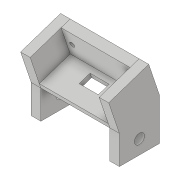
# Autodesk Inventor part: Lidar Sensor Case v3
Saved by Autodesk Inventor 2018.3 (Build 223284000, 284)
## iProperties
Created: 2019-02-04
Part Number: Lidar Sensor Case v3
Material: Generic
Document SubType Name: Modeling
Designer: aye06091
Mass: 24.5359 g
Surface Area: 111.529 cm^2
Volume: 24.5359 cm^3
Density: 1 g/cm^3
Appearance: Default
Author: aye06091
Autodesk Inventor part; units mm, degrees
ref_plane "YZ Plane" through (0, 0, 0) normal (1, 0, 0) x (0, 1, 0)
ref_plane "XZ Plane" through (0, 0, 0) normal (0, 1, 0) x (-1, 0, 0)
sketch "Sketch8" plane through (0, 0, 0) normal (1, 0, 0) x (0, 1, 0)
  line L0 (-3.8078, 7.851) -> (3.0591, -12.6251)
  line L1 (-0.2897, -12.6251) -> (-4.6863, 0.485)
  line L2 (3.0591, -12.6251) -> (-0.2897, -12.6251)
  line L3 (-4.6863, 0.485) -> (-6.818, 6.8414)
  line L4 (-3.8078, 7.851) -> (-6.818, 6.8414)
  point P0 (0, 0)
  dimension "d149" = 21.5968
  dimension "d150" = 3.175
  dimension "d151" = 3.3488
  constraints: 10 end point, 1 horizontal, 1 perpendicular
  measures "d149" distance of L0.start L0.end
  measures "d150" distance of L0.start L3.end
  measures "d151" distance of L0.end L1.start
extrude "Extrusion6" add sketch "Sketch8" along normal blind 45.72
sketch "Sketch11" plane through (0, 0, 0) normal (-1, 0, 0) x (0, 0, 1)
  line L0 (0.485, -4.6863) -> (-12.6251, -0.2897) projected
  line L1 (6.8422, -6.8159) -> (6.835, -6.8159)
  line L2 (-12.6251, -0.2897) -> (0.485, -4.6863)
  line L3 (7.851, -3.8078) -> (-12.6251, 3.0591) projected
  line L4 (13.9082, 14.2533) -> (7.851, -3.808)
  line L5 (7.851, -3.808) -> (-18.639, 5.076)
  line L6 (-18.639, 5.076) -> (-12.5817, 23.1373)
  line L7 (-12.5817, 23.1373) -> (13.9082, 14.2533)
  line L8 (-12.6251, -0.2897) -> (6.8414, -6.818) projected
  line L9 (6.8414, -6.818) -> (7.851, -3.8078) projected
  point P0 (0, 0)
  dimension "d73" = 27.94
  dimension "d76" = 0
  dimension "d88" = 19.05
  constraints: 12 end point, 2 parallel, 2 point on line, 1 perpendicular
  measures "d73" distance of L6.end L4.start
  measures "d76" distance from line of L3 L5.end
  measures "d88" distance of L5.end L6.end
extrude "Extrusion8" add sketch "Sketch11" along normal blind 6.35 contours L3 L5 L6 L7 L4
sketch "Sketch13" plane through (0, -3.8078, 7.851) normal (0, 0.9481042, 0.3179598) x (1, 0, 0)
  line L0 (0, 0) -> (0, 21.5968) projected
  line L1 (16.51, 18.0408) -> (29.21, 18.0408)
  line L2 (29.21, 18.0408) -> (29.21, 10.4208)
  line L3 (29.21, 10.4208) -> (16.51, 10.4208)
  line L4 (16.51, 10.4208) -> (16.51, 18.0408)
  point P0 (0, 8.6543)
  dimension "d55" = 7.62
  dimension "d56" = 12.7
  dimension "d57" = 16.51
  constraints: 8 end point, 2 parallel, 1 horizontal, 1 perpendicular
  measures "d55" distance of L3.end L1.start
  measures "d56" distance of L2.end L3.end
  measures "d57" distance between parallel lines of L0 L4
extrude "Extrusion10" cut sketch "Sketch13" against normal blind 25.4
sketch "Sketch15" plane through (0, 0, 0) normal (1, 0, 0) x (0, 0, -1)
  line L0 (6.5678, 21.1205) -> (12.5883, 23.1395)
  line L1 (12.5883, 23.1395) -> (18.6455, 5.0782)
  line L2 (18.6455, 5.0782) -> (12.6251, 3.0591)
  line L3 (12.6251, 3.0591) -> (6.5678, 21.1205)
  dimension "d67" = 6.35
  dimension "d69" = 0
  dimension "d70" = 0
  dimension "d87" = 19.05
  constraints: 8 end point, 2 parallel, 1 perpendicular
  measures "d67" distance of L0.start L0.end
  measures "d69" distance of point (12.625, 3.059) L2.end
  measures "d70" distance of point (12.625, 3.059) L2.end
  measures "d87" distance of L2.end L0.start
extrude "Extrusion11" add sketch "Sketch15" along normal blind 45.72
sketch "Sketch17" plane through (45.72, 0, 0) normal (1, 0, 0) x (0, 0, -1)
  line L0 (-7.851, -3.808) -> (-13.9082, 14.2533) projected
  line L1 (-7.851, -3.808) -> (-13.9082, 14.2533)
  line L2 (-13.9082, 14.2533) -> (12.5883, 23.1395)
  line L3 (12.5883, 23.1395) -> (18.6456, 5.0782)
  line L4 (18.6456, 5.0782) -> (-7.851, -3.808)
  point P0 (0, 0)
  constraints: 8 end point, 2 parallel, 1 perpendicular
extrude "Extrusion12" add sketch "Sketch17" along normal blind 6.35
sketch "Sketch19" plane through (45.72, 5.0782, -18.6456) normal (0, -0.9481019, -0.3179666) x (1, 0, 0)
  line L0 (0, 6.3501) -> (0, 0.0001) projected
  line L1 (6.35, 27.947) -> (0, 27.947)
  line L2 (0, 27.947) -> (0, 0.0001)
  line L3 (0, 0.0001) -> (6.35, 0.0001)
  line L4 (6.35, 0.0001) -> (6.35, 27.947)
  line L5 (-45.72, 6.3501) -> (0, 6.3501) projected
  line L6 (0, 0.0001) -> (0, 0.0001)
  line L7 (0, 0.0001) -> (0, 6.3501)
  line L8 (0, 6.3501) -> (0, 6.3501)
  line L9 (0, 6.3501) -> (0, 0.0001)
  line L10 (-45.72, 0.007) -> (-52.07, 0.007) projected
  line L11 (-52.07, 0.007) -> (-45.72, 0.007)
  line L12 (-45.72, 0.007) -> (-45.72, 27.947)
  line L13 (-45.72, 27.947) -> (-52.07, 27.947)
  line L14 (-52.07, 27.947) -> (-52.07, 0.007)
  point P0 (-45.72, 19.2926)
  constraints: 24 end point, 6 equal length, 3 horizontal, 3 perpendicular, 1 point on line
extrude "Extrusion13" add sketch "Sketch19" along normal blind 3.175
sketch "Sketch20" plane through (0, 5.0782, -18.6455) normal (0, -0.9481019, -0.3179666) x (1, 0, 0)
  line L0 (45.72, 0) -> (0, 0)
  line L1 (0, 0) -> (0, 6.35)
  line L2 (0, 6.35) -> (45.72, 6.35)
  line L3 (45.72, 6.35) -> (45.72, 0)
  point P0 (0, 19.2926)
  constraints: 8 end point, 2 parallel, 1 horizontal, 1 perpendicular
extrude "Extrusion14" add sketch "Sketch20" along normal blind 3.175
sketch "Sketch21" plane through (0, 0, 0) normal (1, 0, 0) x (0, 0, -1)
  line L0 (19.6485, 2.0658) -> (13.6346, 0.0489) projected
  line L1 (13.6346, 0.0489) -> (12.6251, 3.0591) projected
  line L2 (12.6251, 3.0591) -> (12.6251, -0.2897) projected
  line L3 (12.6251, -0.2897) -> (-6.8414, -6.818) projected
  line L4 (-0.485, -4.6863) -> (-0.485, -4.6865) projected
  line L5 (19.6485, 2.0657) -> (-6.8414, -6.8182) projected
  line L6 (19.6485, 2.0657) -> (19.6485, 2.0658) projected
  line L7 (12.6251, 3.0591) -> (13.6346, 0.0489)
  line L8 (12.6251, -0.2897) -> (13.6346, 0.0489)
  line L9 (12.6251, 3.0591) -> (12.6251, -0.2897)
  point P0 (0, 0)
  point P1 (-6.8415, -6.8181)
  constraints: 6 end point, 2 collinear, 1 perpendicular
extrude "Extrusion15" add sketch "Sketch21" along normal blind 45.72
sketch "Sketch22" plane through (16.51, -1.0818, -10.2631) normal (0, 0.9481042, 0.3179598) x (1, 0, 0)
  line L0 (12.7, -7.62) -> (12.7, 0) projected
  line L1 (12.7, 0) -> (0, 0) projected
  line L2 (0, 0) -> (12.7, 0)
  line L3 (12.7, 0) -> (12.7, -7.62)
  line L4 (12.7, -7.62) -> (0, -7.62)
  line L5 (0, -7.62) -> (0, 0)
  point P0 (-16.51, -9.3866)
  constraints: 8 end point, 2 parallel, 1 horizontal, 1 perpendicular
extrude "Extrusion16" cut sketch "Sketch22" against normal blind 45.72
ref_plane "Work Plane1" through (0, -6.818, 6.8414) normal (0, -1, 0) x (1, 0, 0)
sketch "Sketch31" plane through (0, 21.1205, -6.5678) normal (0, -0.3179666, 0.9481019) x (1, 0, 0)
  line L0 (0, -19.05) -> (45.72, -19.05) projected
  line L1 (8.11, -16.025) -> (37.61, -16.025)
  line L2 (37.61, -16.025) -> (37.61, -13.275)
  line L3 (37.61, -13.275) -> (41.36, -13.275)
  arc A0 (41.36, -13.275) -> (41.36, -5.775) centre (41.36, -9.525) ccw
  line L4 (41.36, -5.775) -> (37.61, -5.775)
  line L5 (37.61, -5.775) -> (37.61, -3.025)
  line L6 (37.61, -3.025) -> (8.11, -3.025)
  line L7 (8.11, -3.025) -> (8.11, -5.775)
  line L8 (8.11, -5.775) -> (4.36, -5.775)
  arc A1 (4.36, -5.775) -> (4.36, -13.275) centre (4.36, -9.525) ccw
  line L9 (4.36, -13.275) -> (8.11, -13.275)
  line L10 (8.11, -13.275) -> (8.11, -16.025)
  circle A2 centre (41.36, -9.525) radius 1.6
  circle A3 centre (4.36, -9.525) radius 1.6
  line L11 (22.86, -3.025) -> (22.86, -16.025)
  line L12 (0, 0) -> (45.72, 0) projected
  line L13 (22.86, 0) -> (22.86, -19.05)
  line L14 (4.36, -9.525) -> (41.36, -9.525)
  line L15 (0, -22.225) -> (0, 0) projected
  line L16 (45.72, -19.05) -> (45.72, 0) projected
  line L17 (0, -9.525) -> (45.72, -9.525)
  point P0 (0, -17.936)
  point P1 (22.86, -9.525)
  point P2 (22.86, -9.525)
  dimension "d132" = 9.525
  constraints: 28 end point, 6 midpoint, 4 centre point, 4 point on circle, 2 point on line, 1 horizontal, 1 perpendicular
  measures "d132" distance between parallel lines of L0 L17
extrude "Extrusion24" cut sketch "Sketch31" against normal through all contours L17 L14 A3 | A3 L14 L17 | L14 L17 A2 | A2 L17 L14
sketch "Sketch32" plane through (52.07, 0, 0) normal (1, 0, 0) x (0, 0, -1)
  line L0 (19.6551, 2.0679) -> (-6.8414, -6.8182) projected
  line L1 (-6.8414, -6.8182) -> (-6.8414, -25.8682)
  line L2 (-6.8414, -25.8682) -> (19.6551, -25.8682)
  line L3 (19.6551, -25.8682) -> (19.6551, 2.0679)
  point P0 (0, 0)
  dimension "d139" = 19.05
  constraints: 6 end point, 2 vertical, 1 parallel
  measures "d139" distance of L0.end L1.end
extrude "Extrusion25" add sketch "Sketch32" against normal up to surface (6.35 mm away)
sketch "Sketch33" plane through (-6.35, 0, 0) normal (-1, 0, 0) x (0, 0, 1)
  line L0 (6.8414, -25.8682) -> (6.8414, -6.8182) projected
  line L1 (-19.6551, -25.8682) -> (6.8414, -25.8682) projected
  line L2 (-19.6551, 2.0679) -> (-19.6551, -25.8682) projected
  line L3 (13.9082, 14.2533) -> (6.8414, -6.8182) projected
  line L4 (-19.6551, 2.0679) -> (6.8414, -6.8182)
  point P0 (0, 0)
  constraints: 2 end point, 1 perpendicular
extrude "Extrusion26" add sketch "Sketch33" against normal up to surface (6.35 mm away)
sketch "Sketch34" plane through (52.07, 0, 0) normal (1, 0, 0) x (0, 0, -1)
  line L0 (-6.8414, -25.8682) -> (-6.8414, -6.8182) projected
  line L1 (19.6551, -25.8682) -> (-6.8414, -25.8682) projected
  circle A0 centre (6.4047, -16.5549) radius 3.302
  point P0 (0, 0)
  dimension "d144" = 6.604
  dimension "d145" = 9.3133
  dimension "d146" = 13.2461
  constraints: 1 centre point
  measures "d144" diameter of A0
  measures "d145" distance from line of L1 A0.centre
  measures "d146" distance from line of L0 A0.centre
extrude "Extrusion27" cut sketch "Sketch34" against normal up to surface (58.42 mm away)
equation "\"d57\" = d58"
equation "\"d58\" = 16.51"
body "Solid3"
